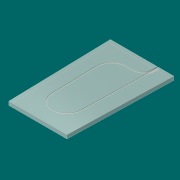
# Autodesk Inventor part: Scintillator Tile
Saved by Autodesk Inventor 2016 (Build 200138000, 138)
## iProperties
Created: 2015-08-14
Part Number: Scintillator Tile
Material: ABS Plastic
Document SubType Name: Modeling
Designer: Cosmic
Density: 1.06 g/cm^3
Appearance: Clear
Author: Cosmic
Autodesk Inventor part; units mm, degrees
ref_plane "YZ Plane" through (0, 0, 0) normal (1, 0, 0) x (0, 1, 0)
ref_plane "XZ Plane" through (0, 0, 0) normal (0, 1, 0) x (-1, 0, 0)
ref_plane "XY Plane" through (0, 0, 0) normal (0, 0, 1) x (1, 0, 0)
sketch "Sketch1" plane through (0, 0, 0) normal (0, 0, 1) x (1, 0, 0)
  line L0 (-55, -94.187) -> (55, -94.187)
  line L1 (55, -94.187) -> (60, 102.7495)
  line L2 (60, 102.7495) -> (-60, 102.7495)
  line L3 (-60, 102.7495) -> (-55, -94.187)
  line L4 (-60, 102.7495) -> (55, -94.187) construction
  line L5 (60, 102.7495) -> (-55, -94.187) construction
  point P0 (0, 0)
  dimension "d136" = 120
  dimension "d138" = 110
  dimension "d139" = 197
  dimension "d140" = 197
  constraints: 12 end point, 2 point on line, 1 horizontal, 1 parallel
  measures "d136" distance of L1.end L2.end
  measures "d138" distance of L0.start L0.end
  measures "d139" distance of L0.end L1.end
  measures "d140" distance of L2.end L0.start
extrude "Extrusion1" add sketch "Sketch1" along normal blind 7
sketch "Sketch22" plane through (0, 0, 0) normal (1, 0, 0) x (0, 1, 0)
  line L0 (102.7495, 0) -> (-94.187, 0) projected
  line L1 (-94.187, 0) -> (-94.187, 7) projected
  line L2 (102.7495, 7) -> (-94.187, 7) projected
  line L3 (102.7495, 0) -> (102.7495, 7) projected
  line L4 (102.7495, 0) -> (102.7495, 7) projected
  line L5 (102.7495, 2.9) -> (98.6495, 2.9)
  line L6 (73.5579, 5.8) -> (-94.187, 5.8)
  line L7 (-94.187, 0) -> (-94.187, 7) projected
  arc A0 (86.1037, 4.35) -> (73.5579, 5.8) centre (73.5579, -49.2) ccw
  arc A1 (86.1037, 4.35) -> (98.6495, 2.9) centre (98.6495, 57.9) ccw
  point P0 (0, 0)
  dimension "d141" = 4.1
  dimension "d142" = 1.2
  dimension "d143" = 55
  dimension "d144" = 55
  dimension "d145" = 4.1
  constraints: 4 end point, 4 point on circle, 3 tangent, 2 centre point, 2 perpendicular, 2 point on line
  measures "d141" distance between parallel lines of L2 L5
  measures "d142" distance between parallel lines of L2 L6
  measures "d143" radius of A0
  measures "d144" radius of A1
  measures "d145" distance of L5.start L5.end
extrude "Extrusion22" cut sketch "Sketch22" along normal through all both and the other way through all contours L5 A1 A0 L6 L1 L2 L3
sketch "Sketch23" plane through (0, 0, 0) normal (0, 0, -1) x (-1, 0, 0)
  line L0 (55, -94.187) -> (-55, -94.187) projected
  line L1 (60, 102.7495) -> (55, -94.187) projected
  line L2 (-60, 102.7495) -> (60, 102.7495) projected
  line L3 (-55, -94.187) -> (-60, 102.7495) projected
  line L4 (-60, 102.7495) -> (60, 102.7495) projected
  line L5 (-30, 102.7495) -> (-30, 58.9322) construction
  line L6 (-30, 58.9322) -> (-27.4911, -39.885) construction
  arc A0 (-27.4911, -39.885) -> (27.4911, -39.885) centre (0, -39.187) ccw construction
  line L7 (27.4911, -39.885) -> (29.6772, 46.2182) construction
  arc A1 (29.6772, 46.2182) -> (2.1861, 74.4162) centre (2.1861, 46.9162) ccw construction
  line L8 (-28.8, 92.7495) -> (-28.8, 102.7495) construction
  line L9 (-55, -94.187) -> (-60, 102.7495) projected
  line L10 (60, 102.7495) -> (55, -94.187) projected
  line L11 (0, -39.187) -> (0, 0) construction
  line L12 (2.1861, 74.4162) -> (-10.4667, 74.4162) construction
  arc A2 (-28.8, 92.7495) -> (-10.4667, 74.4162) centre (-10.4667, 92.7495) ccw construction
  line L13 (-30.6, 102.7495) -> (-30.6, 58.9246)
  line L14 (-30.6, 58.9246) -> (-28.0909, -39.9002)
  arc A3 (-28.0909, -39.9002) -> (28.0909, -39.9002) centre (0, -39.187) ccw
  line L15 (28.0909, -39.9002) -> (30.277, 46.203)
  arc A4 (30.277, 46.203) -> (2.1861, 75.0162) centre (2.1861, 46.9162) ccw
  line L16 (2.1861, 75.0162) -> (-10.4667, 75.0162)
  arc A5 (-28.2, 92.7495) -> (-10.4667, 75.0162) centre (-10.4667, 92.7495) ccw
  line L17 (-28.2, 92.7495) -> (-28.2, 102.7495)
  line L18 (-30.6, 102.7495) -> (-28.2, 102.7495)
  dimension "d148" = 27.5
  dimension "d149" = 27.5
  dimension "d151" = 1.2
  dimension "d152" = 10
  dimension "d153" = 18.3333
  dimension "d154" = 30
  dimension "d155" = 55
  dimension "d156" = 0.6
  constraints: 24 end point, 12 point on circle, 6 centre point, 6 tangent, 3 vertical, 2 parallel, 2 point on line, 1 collinear, 1 horizontal, 1 perpendicular, 7 other
  measures "d148" radius of A0
  measures "d149" radius of A1
  measures "d151" distance between parallel lines of L5 L8
  measures "d152" distance of L8.start L8.end
  measures "d153" radius of A2
  measures "d154" distance of L2.start L5.start
  measures "d155" distance from line of L0 L11.start
  measures "d156" distance between parallel lines of L5 L13
extrude "Extrusion23" add sketch "Sketch23" against normal blind 7 contours L0 L3 L2 L13 L14 A3 L15 A4 L16 A5 L17 L1
sketch "Sketch24" plane through (0, 0, 7) normal (0, 0, 1) x (1, 0, 0)
  line L0 (30.6, 102.7495) -> (30.6, 58.9246) projected
  line L1 (30.6, 58.9246) -> (28.0909, -39.9002) projected
  arc A0 (-28.0909, -39.9002) -> (28.0909, -39.9002) centre (0, -39.187) ccw projected
  line L2 (-28.0909, -39.9002) -> (-30.277, 46.203) projected
  arc A1 (-2.1861, 75.0162) -> (-30.277, 46.203) centre (-2.1861, 46.9162) ccw projected
  line L3 (-2.1861, 75.0162) -> (10.4667, 75.0162) projected
  arc A2 (10.4667, 75.0162) -> (28.2, 92.7495) centre (10.4667, 92.7495) ccw projected
  line L4 (28.2, 92.7495) -> (28.2, 102.7495) projected
  line L5 (28.2, 102.7495) -> (-60, 102.7495) projected
  line L6 (-60, 102.7495) -> (-55, -94.187) projected
  line L7 (-55, -94.187) -> (55, -94.187) projected
  line L8 (55, -94.187) -> (60, 102.7495) projected
  line L9 (60, 102.7495) -> (30.6, 102.7495) projected
  line L10 (10.4667, 73.8162) -> (-2.1861, 73.8162)
  arc A3 (-2.1861, 73.8162) -> (-29.0774, 46.2334) centre (-2.1861, 46.9162) ccw
  line L11 (-29.0774, 46.2334) -> (-26.8913, -39.8698)
  arc A4 (-26.8913, -39.8698) -> (26.8913, -39.8698) centre (0, -39.187) ccw
  line L12 (26.8913, -39.8698) -> (29.4, 58.9398)
  line L13 (29.4, 58.9398) -> (29.4, 92.7495)
  arc A5 (10.4667, 73.8162) -> (29.4, 92.7495) centre (10.4667, 92.7495) ccw
  point P0 (0, 0)
  constraints: 8 end point, 6 point on circle, 3 centre point, 1 tangent, 4 other
extrude "Extrusion24" add sketch "Sketch24" against normal up to surface (7 mm away) contours A5 L13 L12 A4 L11 A3 L10
equation "\"d2\" = ScintillatorThickness"
equation "\"d5\" = OpticalFiberDiameter + 2 * OpticalFiberClearence"
equation "\"d21\" = d5"
equation "\"d22\" = d5"
equation "\"OpticalFiberDiameter\" = 1"
equation "\"ScintillatorThickness\" = 7"
equation "\"OpticalFiberClearence\" = 0.1"
equation "\"SmallTrackDiameter\" = 175"
equation "\"ScintillatorEdgeClearence\" = 3"
equation "\"ScintillatorWidth\" = 145"
equation "\"ScintillatorHeight\" = 145"
equation "\"ShallowTrackDepth\" = 1.2"
equation "\"MPPCClearence\" = 0.075"
equation "\"MPPCSensorClearence\" = 1.45"
equation "\"MPPCSensorOffsett\" = 2.105"
equation "\"MPPCWidth\" = 5.9"
equation "\"MPPCHeight\" = 6.55"
equation "\"FiberEdgeOffsett\" = 5"
equation "\"MPPCDepth\" = 1"
equation "\"LongFiberAngle\" = 30deg"
equation "\"ShortFiberAngle\" = 78deg"
equation "\"LoopLargeTrackRatio\" = 1.1"
equation "\"LoopSmallTrackDiameter\" = 55"
equation "\"FiberSensorClerence\" = 0.5"
equation "\"MountingScrewOffsett\" = 12.5"
equation "\"MountingScrewDepth\" = 4"
equation "\"DeepTrackDepth\" = 4.1"
body "Solid1"
